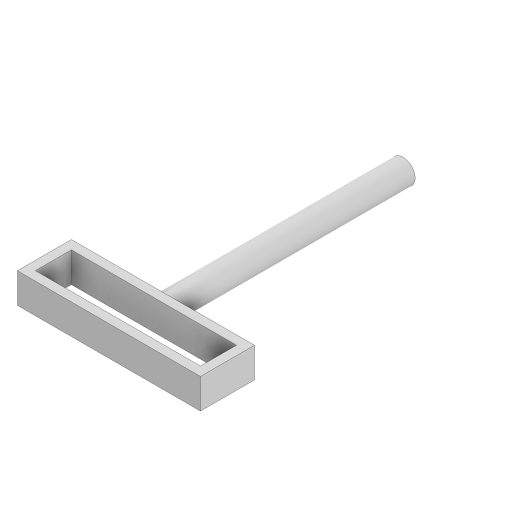
# Autodesk Inventor part: YUGO
Saved by Autodesk Inventor 2024 (Build 280153000, 153)
## iProperties
Created: 2024-06-30
Part Number: YUGO
Material: Generic
Document SubType Name: Modeling
Designer: Jhuliams
Density: 1 g/cm^3
Appearance: Default
Author: Jhuliams
Autodesk Inventor part; units mm, degrees
ref_plane "YZ Plane" through (0, 0, 0) normal (1, 0, 0) x (0, 1, 0)
ref_plane "XZ Plane" through (0, 0, 0) normal (0, 1, 0) x (-1, 0, 0)
ref_plane "XY Plane" through (0, 0, 0) normal (0, 0, 1) x (1, 0, 0)
sketch "Sketch1" plane through (0, 0, 0) normal (0, 1, 0) x (-1, 0, 0)
  line L0 (27.5, 6) -> (-27.5, 6)
  line L1 (-27.5, 6) -> (-27.5, -6)
  line L2 (-27.5, -6) -> (27.5, -6)
  line L3 (27.5, -6) -> (27.5, 6)
  line L4 (27.5, 6) -> (-27.5, -6) construction
  line L5 (-27.5, 6) -> (27.5, -6) construction
  line L6 (30.5, -9) -> (-30.5, -9)
  line L7 (-30.5, -9) -> (-30.5, 9)
  line L8 (-30.5, 9) -> (30.5, 9)
  line L9 (30.5, 9) -> (30.5, -9)
  point P0 (0, 0)
  dimension "d0" = 55
  dimension "d1" = 12
  dimension "d2" = 3
  constraints: 20 end point, 4 parallel, 2 midpoint, 2 perpendicular, 1 horizontal, 3 other
  measures "d0" distance of L2.end L1.end
  measures "d1" distance of L1.end L0.end
  measures "d2" distance between parallel lines of L2 L6
extrude "Extrusion1" add sketch "Sketch1" along normal blind 10
sketch "Sketch2" plane through (30.5, 0, -9) normal (0, 0, -1) x (-1, 0, 0)
  line L0 (30.5, 0) -> (30.5, 5)
  circle A0 centre (30.5, 5) radius 4
  dimension "d5" = 5
  dimension "d6" = 8
  constraints: 2 end point, 1 centre point, 1 coincident, 1 vertical
  measures "d5" distance of L0.start L0.end
  measures "d6" diameter of A0
extrude "Extrusion2" add sketch "Sketch2" along normal blind 80
body "Solid1"
